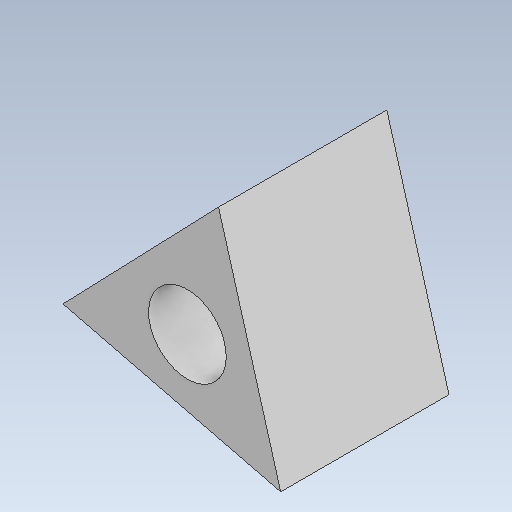
# Autodesk Inventor part: HandlePotAttachmentGear
Saved by Autodesk Inventor 2021 (Build 250183000, 183)
## iProperties
Created: 2021-03-20
Part Number: HandlePotAttachmentGear
Material: Generic
Document SubType Name: Modeling
Designer: ben
Density: 1 g/cm^3
Appearance: Default
Author: ben
Autodesk Inventor part; units mm, degrees
ref_plane "YZ Plane" through (0, 0, 0) normal (1, 0, 0) x (0, 1, 0)
ref_plane "XZ Plane" through (0, 0, 0) normal (0, 1, 0) x (-1, 0, 0)
ref_plane "XY Plane" through (0, 0, 0) normal (0, 0, 1) x (1, 0, 0)
sketch "Sketch1" plane through (0, 0, 0) normal (0, 0, 1) x (1, 0, 0)
  line L0 (-1.6614, 3.5785) -> (-2.5268, 3.4417) projected
  line L1 (-2.0457, 4.3659) -> (-1.6614, 3.5785) projected
  line L2 (-1.1857, 4.1985) -> (-2.0457, 4.3659) projected
  line L3 (-1.2776, 5.0698) -> (-1.1857, 4.1985) projected
  line L4 (-0.5267, 4.6183) -> (-1.2776, 5.0698) projected
  line L5 (-0.315, 5.4685) -> (-0.5267, 4.6183) projected
  line L6 (-0.5267, 4.6183) -> (-0.315, 5.4685) projected
  arc A0 (-0.315, 5.4685) -> (-1.2776, 5.0698) centre (0.3343, 2.5396) ccw projected
  line L7 (-1.2776, 5.0698) -> (-0.5267, 4.6183) projected
  arc A1 (-1.2776, 5.0698) -> (-2.0457, 4.3659) centre (0.3343, 2.5396) ccw projected
  line L8 (-1.1857, 4.1985) -> (-1.2776, 5.0698) projected
  arc A2 (-1.2776, 5.0698) -> (-2.0457, 4.3659) centre (0.3343, 2.5396) ccw projected
  line L9 (-2.0457, 4.3659) -> (-1.1857, 4.1985) projected
  line L10 (-2.5268, 3.4417) -> (-1.6614, 3.5785) projected
  line L11 (-1.6614, 3.5785) -> (-2.0457, 4.3659) projected
  arc A3 (-2.0457, 4.3659) -> (-2.5268, 3.4417) centre (0.3343, 2.5396) ccw projected
  line L12 (0.2362, 4.7875) -> (0.7259, 5.5139) projected
  arc A4 (0.7259, 5.5139) -> (-0.315, 5.4685) centre (0.3343, 2.5396) ccw projected
  line L13 (-0.315, 5.4685) -> (0.2362, 4.7875) projected
  line L14 (1.0109, 4.6855) -> (1.7196, 5.2006) projected
  arc A5 (1.7196, 5.2006) -> (0.7259, 5.5139) centre (0.3343, 2.5396) ccw projected
  line L15 (0.7259, 5.5139) -> (1.0109, 4.6855) projected
  line L16 (1.7196, 5.2006) -> (1.7041, 4.3247) projected
  line L17 (1.7041, 4.3247) -> (2.5462, 4.5664) projected
  arc A6 (2.5462, 4.5664) -> (1.7196, 5.2006) centre (0.3343, 2.5396) ccw projected
  line L18 (2.5462, 4.5664) -> (2.232, 3.7485) projected
  line L19 (2.232, 3.7485) -> (3.106, 3.6877) projected
  arc A7 (3.106, 3.6877) -> (2.5462, 4.5664) centre (0.3343, 2.5396) ccw projected
  line L20 (3.106, 3.6877) -> (2.531, 3.0266) projected
  line L21 (2.531, 3.0266) -> (3.3315, 2.6705) projected
  arc A8 (3.3315, 2.6705) -> (3.106, 3.6877) centre (0.3343, 2.5396) ccw projected
  line L22 (-2.6628, 2.4087) -> (-2.632, 2.4258) projected
  line L23 (-2.632, 2.4258) -> (3.1702, 1.662) projected
  line L24 (3.1702, 1.662) -> (3.1955, 1.6375) projected
  arc A9 (3.1955, 1.6375) -> (3.3315, 2.6705) centre (0.3343, 2.5396) ccw projected
  line L25 (3.3315, 2.6705) -> (3.3007, 2.6534) projected
  line L26 (3.3007, 2.6534) -> (-2.5015, 3.4173) projected
  line L27 (-2.5015, 3.4173) -> (-2.5268, 3.4417) projected
  arc A10 (-2.5268, 3.4417) -> (-2.6628, 2.4087) centre (0.3343, 2.5396) ccw projected
  line L28 (3.1955, 1.6375) -> (2.3301, 1.5007) projected
  line L29 (2.3301, 1.5007) -> (2.7144, 0.7133) projected
  arc A11 (2.7144, 0.7133) -> (3.1955, 1.6375) centre (0.3343, 2.5396) ccw projected
  line L30 (2.7144, 0.7133) -> (1.8544, 0.8807) projected
  line L31 (1.8544, 0.8807) -> (1.9462, 0.0094) projected
  arc A12 (1.9462, 0.0094) -> (2.7144, 0.7133) centre (0.3343, 2.5396) ccw projected
  line L32 (1.1954, 0.4609) -> (0.9837, -0.3893) projected
  arc A13 (0.9837, -0.3893) -> (1.9462, 0.0094) centre (0.3343, 2.5396) ccw projected
  line L33 (1.9462, 0.0094) -> (1.1954, 0.4609) projected
  line L34 (0.4325, 0.2917) -> (-0.0572, -0.4347) projected
  arc A14 (-0.0572, -0.4347) -> (0.9837, -0.3893) centre (0.3343, 2.5396) ccw projected
  line L35 (0.9837, -0.3893) -> (0.4325, 0.2917) projected
  line L36 (-0.3422, 0.3937) -> (-1.0509, -0.1214) projected
  arc A15 (-1.0509, -0.1214) -> (-0.0572, -0.4347) centre (0.3343, 2.5396) ccw projected
  line L37 (-0.0572, -0.4347) -> (-0.3422, 0.3937) projected
  line L38 (-1.0354, 0.7546) -> (-1.8775, 0.5128) projected
  arc A16 (-1.8775, 0.5128) -> (-1.0509, -0.1214) centre (0.3343, 2.5396) ccw projected
  line L39 (-1.0509, -0.1214) -> (-1.0354, 0.7546) projected
  line L40 (-1.5633, 1.3307) -> (-2.4373, 1.3916) projected
  arc A17 (-2.4373, 1.3916) -> (-1.8775, 0.5128) centre (0.3343, 2.5396) ccw projected
  line L41 (-1.8775, 0.5128) -> (-1.5633, 1.3307) projected
  line L42 (-2.4373, 1.3916) -> (-1.8623, 2.0526) projected
  line L43 (-1.8623, 2.0526) -> (-2.6628, 2.4087) projected
  arc A18 (-2.6628, 2.4087) -> (-2.4373, 1.3916) centre (0.3343, 2.5396) ccw projected
  line L44 (7.5399, -4.3947) -> (-9.2738, -0.2334)
  line L45 (-9.2738, -0.2334) -> (2.7369, 12.247)
  line L46 (2.7369, 12.247) -> (7.5399, -4.3947)
  dimension "d0" = 17.321
  constraints: 6 end point, 1 coincident, 7 other
  measures "d0" distance of L45.end L44.start
ref_plane "Work Plane1" through (-2.6657, -0.4604, -13) normal (0, 0, -1) x (0, 1, 0)
extrude "Extrusion1" add sketch "Sketch1" against normal up to surface (13 mm away)
body "Solid1"
